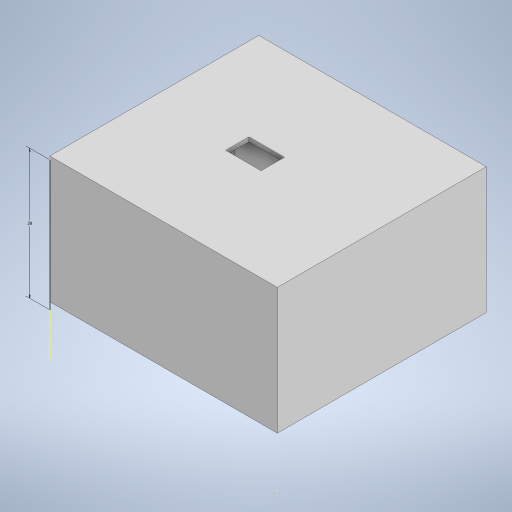
# Autodesk Inventor part: Część6
Saved by Autodesk Inventor 2024.3 (Build 283343000, 343)
## iProperties
Created: 2024-07-18
Part Number: Część6
Material: Ogólny
Document SubType Name: Modeling
Designer: User
Density: 1 g/cm^3
Appearance: Domyślna
Author: User
Autodesk Inventor part; units mm, degrees
ref_plane "YZ Plane" through (0, 0, 0) normal (1, 0, 0) x (0, 1, 0)
ref_plane "XZ Plane" through (0, 0, 0) normal (0, 1, 0) x (-1, 0, 0)
ref_plane "XY Plane" through (0, 0, 0) normal (0, 0, 1) x (1, 0, 0)
sketch "Szkic1" plane through (0, 0, 0) normal (0, 1, 0) x (-1, 0, 0)
  line L0 (0, 0) -> (49, 0)
  line L1 (49, 0) -> (49, -45)
  line L2 (49, -45) -> (0, -45)
  line L3 (0, -45) -> (0, 0)
  line L4 (49, 0) -> (49, 3)
  line L5 (49, 3) -> (52, 3)
  line L6 (0, -45) -> (0, -48)
  line L7 (0, -48) -> (-3, -48)
  line L8 (-3, -48) -> (52, -48)
  line L9 (52, -48) -> (52, 3)
  line L10 (52, 3) -> (-3, 3)
  line L11 (-3, 3) -> (-3, -48)
  line L12 (0, -48) -> (-29.5685, -48)
  line L13 (-29.5685, -48) -> (-29.5685, 3)
  line L14 (-29.5685, 3) -> (0, 3)
  line L15 (0, 3) -> (0, -48)
  line L16 (-3, -45) -> (-29.5685, -45)
  line L17 (-3, 0) -> (-29.5685, 0)
  line L18 (-3, 0) -> (0, 0)
  line L19 (0, -45) -> (-3, -45)
  line L20 (-3, -45) -> (-3, -48)
  line L21 (0, -48) -> (0, -45)
  line L22 (0, -48) -> (-3, -48)
  dimension "d0" = 49
  dimension "d1" = 45
  dimension "d2" = 3
  dimension "d3" = 3
  dimension "d4" = 3
  dimension "d5" = 3
  constraints: 46 end point, 8 perpendicular, 6 parallel, 4 horizontal, 4 point on line, 3 collinear, 2 vertical
  measures "d0" distance of L1.end L2.end
  measures "d1" distance of L0.end L1.end
  measures "d2" distance of L0.end L4.end
  measures "d3" distance of L4.end L5.end
  measures "d4" distance of L2.end L6.end
  measures "d5" distance of L6.end L7.end
extrude "Wyciągnięcie proste1" add sketch "Szkic1" along normal blind 37.2 contours L0 L1 L2 L3 | L3 L19 L11 L18 | L11 L16 L13 L17
sketch "Szkic2" plane through (0, 0, 0) normal (0, -1, 0) x (1, 0, 0)
  line L0 (-49, 0) -> (0, 0) projected
  line L1 (-24.5, 0) -> (-24.5, -45)
  line L2 (0, -45) -> (-49, -45) projected
  line L3 (-49, -45) -> (-49, 0) projected
  line L4 (-49, -22.5) -> (0, -22.5)
  line L5 (0, 0) -> (0, -45) projected
  circle A0 centre (-24.5, -22.5) radius 2.85
  circle A1 centre (-24.5, -22.5) radius 3
  dimension "d8" = 5.7
  dimension "d27" = 6
  constraints: 5 midpoint, 4 end point, 2 centre point, 1 coincident
  measures "d8" diameter of A0
  measures "d27" diameter of A1
extrude "Wyciągnięcie proste2" cut sketch "Szkic2" against normal through all contours A1 L4 A0 L1 | L1 A0 L4 A1 | L4 A0 L1 A1 | A0 L4 L1 | L1 L4 A0 | A1 L1 A0 L4 | L4 L1 A0 | L4 A0 L1
sketch "Szkic3" plane through (0, 0, 0) normal (0, -1, 0) x (1, 0, 0)
  circle A0 centre (-24.5, -22.5) radius 2.85 projected
  line L0 (-24.5, -22.5) -> (-37.8, -22.5)
  line L1 (-24.5, -22.5) -> (9, -22.5)
  line L2 (-37.8, -22.5) -> (9, -22.5)
  line L3 (9, -22.5) -> (9, -32.4)
  line L4 (9, -32.4) -> (-37.8, -32.4)
  line L5 (-37.8, -32.4) -> (-37.8, -22.5)
  line L6 (9, -22.5) -> (-37.8, -22.5)
  line L7 (-37.8, -22.5) -> (-37.8, -13.6)
  line L8 (-37.8, -13.6) -> (9, -13.6)
  line L9 (9, -13.6) -> (9, -22.5)
  line L10 (9, -32.4) -> (-37.8, -32.4)
  line L11 (9, -32.4) -> (13, -32.4)
  line L12 (-37.8, -13.6) -> (-41.8, -13.6)
  line L13 (13, -32.4) -> (13, -32.9)
  line L14 (-41.8, -13.6) -> (-41.8, -13)
  line L15 (13, -32.4) -> (13, -33)
  line L16 (-41.8, -13) -> (-42.5873, -13)
  line L17 (13, -33) -> (13.5, -33)
  line L18 (13.5, -33) -> (-42.5873, -33)
  line L19 (-42.5873, -33) -> (-42.5873, -13)
  line L20 (-42.5873, -13) -> (13.5, -13)
  line L21 (13.5, -13) -> (13.5, -33)
  line L22 (13.5, -13) -> (-6.5, -13)
  line L23 (-6.5, -13) -> (-6.5, -32.4)
  line L24 (-6.5, -32.4) -> (13.5, -32.4)
  line L25 (13.5, -32.4) -> (13.5, -13)
  line L26 (-37.8, -22.5) -> (-6.5, -22.5)
  line L27 (-6.5, -22.5) -> (-6.5, -16.35)
  line L28 (-6.5, -16.35) -> (-37.8, -16.35)
  line L29 (-37.8, -16.35) -> (-37.8, -22.5)
  line L30 (-37.8, -22.5) -> (-6.5, -22.5)
  line L31 (-6.5, -22.5) -> (-6.5, -28.65)
  line L32 (-6.5, -28.65) -> (-37.8, -28.65)
  line L33 (-37.8, -28.65) -> (-37.8, -22.5)
  line L34 (-6.5, -16.35) -> (-5.5, -16.35)
  line L35 (-5.5, -16.35) -> (-5.5, -28.65)
  line L36 (-5.5, -28.65) -> (-6.5, -28.65)
  line L37 (-6.5, -28.65) -> (-6.5, -16.35)
  line L38 (-37.8, -22.5) -> (-26.4, -22.5)
  line L39 (-24.5, -22.5) -> (-26.9, -22.5)
  circle A1 centre (-26.9, -22.5) radius 2.4
  point P0 (0, 0)
  dimension "d21" = 4
  dimension "d22" = 4
  dimension "d23" = 0.5
  dimension "d24" = 0.6
  dimension "d25" = 0.6
  dimension "d26" = 0.5
  dimension "d28" = 20
  dimension "d29" = 6.15
  dimension "d30" = 6.15
  dimension "d31" = 1
  dimension "d32" = 11.4
  dimension "d33" = 2.4
  dimension "d34" = 4.8
  constraints: 80 end point, 15 equal length, 13 horizontal, 7 perpendicular, 7 point on line, 2 vertical, 1 centre point, 1 coincident
  measures "d21" distance of L3.end L11.end
  measures "d22" distance of L7.end L12.end
  measures "d23" distance of L11.end L13.end
  measures "d24" distance of L12.end L14.end
  measures "d25" distance of L11.end L15.end
  measures "d26" distance of L15.end L17.end
  measures "d28" distance of L24.end L23.end
  measures "d29" distance of L27.end L26.end
  measures "d30" distance of L30.end L31.end
  measures "d31" distance of L35.end L36.end
  measures "d32" distance of L6.end L38.end
  measures "d33" distance of L0.start L39.end
  measures "d34" diameter of A1
extrude "Wyciągnięcie proste3" cut sketch "Szkic3" against normal blind 37 contours L1 L23 L32 L5 L0 A1 A0 | A0 A1 L0 L7 L28 L23 L1 | A0 L0 A1 | A1 L0 A0 | L23 L34 L35 L1 | L1 L35 L36 L23 | L24 L21 L17 L15 L13 picked at (-27.9524, -22.0946) picked at (-27.9524, -22.9054)
sketch "Szkic4" plane through (0, 0, 0) normal (0, -1, 0) x (1, 0, 0)
  line L0 (-49, -45) -> (-49, 0) projected
  line L1 (-37.8, -28.65) -> (-37.8, -16.35) projected
  line L2 (-49, -22.5) -> (-37.8, -22.5)
  line L3 (-37.8, -22.5) -> (-37.8, -17.5)
  line L4 (-37.8, -17.5) -> (-49, -17.5)
  line L5 (-49, -17.5) -> (-49, -22.5)
  line L6 (-49, -22.5) -> (-37.8, -22.5)
  line L7 (-37.8, -22.5) -> (-37.8, -27.5)
  line L8 (-37.8, -27.5) -> (-49, -27.5)
  line L9 (-49, -27.5) -> (-49, -22.5)
  point P0 (0, 0)
  point P1 (-37.8, -32.4)
  point P2 (-37.8, -13.6)
  dimension "d17" = 5
  dimension "d18" = 5
  constraints: 16 end point, 4 parallel, 2 horizontal, 2 perpendicular, 2 point on line, 1 midpoint
  measures "d17" distance of L3.end L2.end
  measures "d18" distance of L6.end L7.end
extrude "Wyciągnięcie proste4" cut sketch "Szkic4" against normal blind 10
sketch "Szkic5" plane through (0, 37, 0) normal (0, -1, 0) x (1, 0, 0)
  line L0 (-37.8, -28.65) -> (-37.8, -16.35) projected
  line L1 (-37.8, -22.5) -> (-26.3, -22.5)
  line L2 (-26.3, -22.5) -> (-28.7, -22.5)
  circle A0 centre (-28.7, -22.5) radius 2.4
  point P0 (0, 0)
  dimension "d35" = 11.5
  dimension "d36" = 2.4
  dimension "d37" = 4.8
  constraints: 4 end point, 1 centre point, 1 coincident, 1 horizontal, 1 midpoint, 1 point on line
  measures "d35" distance of L1.start L1.end
  measures "d36" distance of L1.end L2.end
  measures "d37" diameter of A0
extrude "Wyciągnięcie proste5" cut sketch "Szkic5" against normal blind 37
sketch "Szkic6" plane through (0, 37, 0) normal (0, -1, 0) x (1, 0, 0)
  arc A0 (-26.9857, -20.8203) -> (-26.9857, -24.1797) centre (-28.7, -22.5) ccw projected
  circle A1 centre (-28.7, -22.5) radius 2.4
  arc A2 (-26.9857, -24.1797) -> (-26.9857, -20.8203) centre (-24.5, -22.5) ccw projected
  circle A3 centre (-24.5, -22.5) radius 3
  point P0 (0, 0)
  constraints: 2 centre point, 2 coincident
extrude "Wyciągnięcie proste6" add sketch "Szkic6" against normal blind 0.2 contours A2 A1
sketch "Szkic7" plane through (0, 0, 0) normal (0, -1, 0) x (1, 0, 0)
  line L0 (-49, 0) -> (29.5685, 0) projected
  line L1 (-49, 0) -> (0, 0)
  line L2 (29.5685, 0) -> (29.5685, -45) projected
  line L3 (0, 0) -> (29.5685, 0)
  line L4 (29.5685, 0) -> (29.5685, -45)
  line L5 (29.5685, -45) -> (0, -45)
  line L6 (0, -45) -> (0, 0)
  dimension "d42" = 49
  constraints: 10 end point, 2 parallel, 1 collinear, 1 horizontal, 1 perpendicular
  measures "d42" distance of L0.start L1.end
extrude "Wyciągnięcie proste7" cut sketch "Szkic7" against normal through all
sketch "Szkic8" plane through (0, 0, 0) normal (0, -1, 0) x (1, 0, 0)
  line L0 (-49, -45) -> (-49, 0) projected
  line L1 (0, 0) -> (0, -45) projected
  line L2 (-49, 0) -> (0, 0)
  line L3 (0, 0) -> (0, -45)
  line L4 (0, -45) -> (-49, -45)
  line L5 (-49, -45) -> (-49, 0)
  constraints: 8 end point, 2 parallel, 1 horizontal, 1 perpendicular
sketch "Szkic9" plane through (-49, 0, 0) normal (0, 0, 1) x (1, 0, 0)
  line L0 (0, 37.2) -> (0, 9.2)
  line L1 (0, 0) -> (0, 37.2) projected
  point P0 (49, 0)
  dimension "d45" = 28
  constraints: 2 end point, 1 point on line
  measures "d45" distance of L0.start L0.end
extrude "Wyciągnięcie proste8" cut sketch "Szkic8" against normal blind 9.2
sketch "Szkic10" plane through (0, 10, 0) normal (0, -1, 0) x (1, 0, 0)
  line L0 (-49, -45) -> (-49, -27.5) projected
  line L1 (-37.8, -28.65) -> (-37.8, -16.35) projected
  line L2 (-49, -27.5) -> (-37.8, -27.5)
  line L3 (-37.8, -27.5) -> (-37.8, -17.4794)
  line L4 (-37.8, -17.4794) -> (-49, -17.4794)
  line L5 (-49, -17.4794) -> (-49, -27.5)
  point P0 (0, 0)
  constraints: 8 end point, 2 parallel, 1 horizontal, 1 perpendicular, 1 point on line
extrude "Wyciągnięcie proste9" cut sketch "Szkic10" against normal blind 5.55
sketch "Szkic11" plane through (0, 37.2, 0) normal (0, 1, 0) x (1, 0, 0)
  circle A0 centre (-28.7, 22.5) radius 2.4 projected
  circle A1 centre (-28.7, 22.5) radius 2.4
  line L0 (-49, 45) -> (-49, 27.5) projected
  line L1 (0, 0) -> (-49, 0)
  line L2 (-49, 0) -> (-49, 45)
  line L3 (-49, 45) -> (0, 45)
  line L4 (0, 45) -> (0, 0)
  constraints: 8 end point, 2 parallel, 1 centre point, 1 coincident, 1 horizontal, 1 perpendicular
extrude "Wyciągnięcie proste10" add sketch "Szkic11" along normal blind 1
sketch "Szkic12" plane through (0, 9.2, 0) normal (0, -1, 0) x (1, 0, 0)
  line L0 (0, -45) -> (-49, -45) projected
  line L1 (-49, 0) -> (0, 0)
  line L2 (0, 0) -> (0, -45)
  line L3 (0, -45) -> (-49, -45)
  line L4 (-49, -45) -> (-49, 0)
  constraints: 8 end point, 2 parallel, 1 horizontal, 1 perpendicular
extrude "Wyciągnięcie proste11" cut sketch "Szkic12" against normal blind 1.5
sketch "Szkic13" plane through (0, 38.2, 0) normal (0, 1, 0) x (1, 0, 0)
  line L0 (-49, 45) -> (-49, 0) projected
  line L1 (-49, 22.5) -> (-26, 22.5)
  line L2 (-26, 22.5) -> (-28.4, 22.5)
  circle A0 centre (-28.4, 22.5) radius 2.5
  circle A1 centre (-26, 22.5) radius 2.5
  circle A2 centre (-27.2, 22.5) radius 2.5
  line L3 (-23.5, 20) -> (-31.1111, 20)
  line L4 (-31.1111, 20) -> (-31.1111, 25)
  line L5 (-31.1111, 25) -> (-23.5, 25)
  line L6 (-23.5, 25) -> (-23.5, 20)
  point P0 (0, 0)
  dimension "d54" = 23
  dimension "d55" = 2.4
  dimension "d56" = 5
  dimension "d57" = 5
  dimension "d58" = 5
  constraints: 12 end point, 3 centre point, 2 coincident, 2 horizontal, 2 midpoint, 2 parallel, 1 perpendicular, 1 point on line
  measures "d54" distance of L1.start L1.end
  measures "d55" distance of L1.end L2.end
  measures "d56" diameter of A0
  measures "d57" diameter of A1
  measures "d58" diameter of A2
extrude "Wyciągnięcie proste12" cut sketch "Szkic13" against normal blind 1.5
sketch "Szkic14" plane through (0, 38.2, 0) normal (0, 1, 0) x (1, 0, 0)
  line L0 (-54.5366, 52.5987) -> (6.0904, 52.5987)
  line L1 (6.0904, 52.5987) -> (6.0904, -5.7213)
  line L2 (6.0904, -5.7213) -> (-54.5366, -5.7213)
  line L3 (-54.5366, -5.7213) -> (-54.5366, 52.5987)
  point P0 (0, 0)
  constraints: 8 end point, 2 parallel, 1 horizontal, 1 perpendicular
extrude "Wyciągnięcie proste13" cut sketch "Szkic14" against normal blind 0.3
